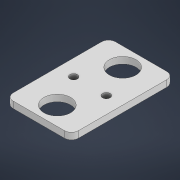
# Autodesk Inventor part: Bearing Bushing
Saved by Autodesk Inventor 2022 (Build 260153000, 153)
## iProperties
Created: 2022-01-18
Part Number: Bearing Bushing
Material: Generic
Document SubType Name: Modeling
Designer: izack
Density: 1 g/cm^3
Appearance: Default
Author: izack
## iProperties of the stored document Bearing Bushing_3DPrint.ipt
Part Number: Bearing Bushing_3DPrint
Material: Generic
Document SubType Name: Modeling
Designer: izack
Appearance: Default
Author: izack
Autodesk Inventor part; units mm, degrees
ref_plane "YZ Plane" through (0, 0, 0) normal (1, 0, 0) x (0, 1, 0)
ref_plane "XZ Plane" through (0, 0, 0) normal (0, 1, 0) x (-1, 0, 0)
ref_plane "XY Plane" through (0, 0, 0) normal (0, 0, 1) x (1, 0, 0)
sketch "Sketch1" plane through (0, 0, 0) normal (0, 1, 0) x (-1, 0, 0)
  line L0 (0, 0) -> (15, 0)
  line L1 (15, 0) -> (15, -15)
  line L2 (15, -15) -> (0, -15)
  line L3 (0, -15) -> (0, 0)
  circle A0 centre (7.5, -22.5) radius 6.1214
  line L4 (15, -7.5) -> (0, -7.5) construction
  circle A1 centre (7.5, 7.5) radius 6.1214
  line L5 (15, 0) -> (0, 0)
  line L6 (0, 3.175) -> (0, 11.825)
  line L7 (3.175, 15) -> (11.825, 15)
  line L8 (15, 11.825) -> (15, 3.175)
  line L9 (15, -15) -> (0, -15)
  line L10 (0, -18.175) -> (0, -26.825)
  line L11 (3.175, -30) -> (11.825, -30)
  line L12 (15, -26.825) -> (15, -18.175)
  arc A2 (15, 11.825) -> (11.825, 15) centre (11.825, 11.825) ccw
  arc A3 (3.175, 15) -> (0, 11.825) centre (3.175, 11.825) ccw
  arc A4 (0, -26.825) -> (3.175, -30) centre (3.175, -26.825) ccw
  arc A5 (11.825, -30) -> (15, -26.825) centre (11.825, -26.825) ccw
  line L13 (18.175, 0) -> (19.325, 0)
  line L14 (22.5, -3.175) -> (22.5, -11.825)
  line L15 (19.325, -15) -> (18.175, -15)
  line L16 (15, -15) -> (15, 0)
  line L17 (-3.175, -15) -> (-4.325, -15)
  line L18 (-7.5, -11.825) -> (-7.5, -3.175)
  line L19 (-4.325, 0) -> (-3.175, 0)
  line L20 (0, 0) -> (0, -15)
  circle A6 centre (0, -7.5) radius 1.75
  circle A7 centre (15, -7.5) radius 1.75
  arc A8 (22.5, -3.175) -> (19.325, 0) centre (19.325, -3.175) ccw
  arc A9 (19.325, -15) -> (22.5, -11.825) centre (19.325, -11.825) ccw
  arc A10 (-7.5, -11.825) -> (-4.325, -15) centre (-4.325, -11.825) ccw
  arc A11 (-4.325, 0) -> (-7.5, -3.175) centre (-4.325, -3.175) ccw
  arc A12 (-3.175, 0) -> (0, 3.175) centre (-3.175, 3.175) ccw
  arc A13 (0, -18.175) -> (-3.175, -15) centre (-3.175, -18.175) ccw
  arc A14 (18.175, -15) -> (15, -18.175) centre (18.175, -18.175) ccw
  arc A15 (15, 3.175) -> (18.175, 0) centre (18.175, 3.175) ccw
  line L21 (19.325, -30.995) -> (-4.325, -30.995)
  line L22 (-7.5, -27.82) -> (-7.5, 12.82)
  line L23 (-4.325, 15.995) -> (19.325, 15.995)
  line L24 (22.5, 12.82) -> (22.5, -27.82)
  arc A16 (-4.325, 15.995) -> (-7.5, 12.82) centre (-4.325, 12.82) ccw
  arc A17 (22.5, 12.82) -> (19.325, 15.995) centre (19.325, 12.82) ccw
  arc A18 (19.325, -30.995) -> (22.5, -27.82) centre (19.325, -27.82) ccw
  arc A19 (-7.5, -27.82) -> (-4.325, -30.995) centre (-4.325, -27.82) ccw
  point P0 (0, 15)
  point P1 (15, 15)
  point P2 (0, -30)
  point P3 (15, -30)
  point P4 (22.5, -15)
  point P5 (22.5, 0)
  point P6 (-7.5, 0)
  point P7 (-7.5, -15)
  point P8 (-7.5, 15.995)
  point P9 (-7.5, -30.995)
  point P10 (-7.5, -7.5)
  dimension "d0" = 15
  dimension "d1" = 15
  dimension "d2" = 12.2428
  dimension "d3" = 7.5
  dimension "d4" = 7.5
  dimension "d5" = 15
  dimension "d6" = 15
  dimension "d7" = 15
  dimension "d8" = 15
  dimension "d9" = 3.175
  dimension "d10" = 7.5
  dimension "d11" = 15
  dimension "d12" = 7.5
  dimension "d13" = 15
  dimension "d14" = 3.5
  dimension "d15" = 3.5
  dimension "d16" = 3.175
  dimension "d19" = 46.99
  dimension "d20" = 3.175
  constraints: 50 end point, 32 point on circle, 32 tangent, 29 point on line, 20 centre point, 13 equal radius, 12 parallel, 6 horizontal, 6 perpendicular, 3 midpoint, 2 coincident, 1 symmetric about line, 1 other
  measures "d0" distance of L1.end L2.end
  measures "d1" distance of L0.end L1.end
  measures "d2" diameter of A0
  measures "d3" distance from line of L3 A0.centre
  measures "d4" distance from line of A0.centre L2
  measures "d5" distance of point (0, 15) point (15, 15)
  measures "d6" distance of L5.end point (0, 15)
  measures "d7" distance of point (15, -30) point (0, -30)
  measures "d8" distance of point (0, -30) L9.end
  measures "d9" radius of A2
  measures "d10" distance of point (22.5, -15) L16.start
  measures "d11" distance of point (22.5, 0) point (22.5, -15)
  measures "d12" distance of point (-7.5, 0) L20.start
  measures "d13" distance of point (-7.5, -15) point (-7.5, 0)
  measures "d14" diameter of A6
  measures "d15" diameter of A7
  measures "d16" radius of A8
  measures "d19" distance of point (-7.5, -30.995) point (-7.5, 15.995)
  measures "d20" radius of A16
extrude "Extrusion1" add sketch "Sketch1" along normal blind 3 contours L0 L1 A7 L2 L3 A6 | A12 L19 A11 L22 A16 L23 A17 L24 A8 L13 A15 L8 A2 L7 A3 L6 | L6 A3 L7 A2 L8 A15 L13 A8 L14 A9 L15 A14 L12 A5 L11 A4 L10 A13 L17 A10 L18 A11 L19 A12 | A10 L17 A13 L10 A4 L11 A5 L12 A14 L15 A9 L24 A18 L21 A19 L22
body "Solid1"
